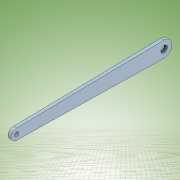
# Autodesk Inventor part: Transmision_Sup
Saved by Autodesk Inventor 2022 (Build 260153000, 153)
## iProperties
Created: 2022-02-14
Part Number: Transmision_Sup
Material: Genérico
Document SubType Name: Modeling
Designer: Marco
Density: 1 g/cm^3
Appearance: Azul acero
Author: Marco
Autodesk Inventor part; units mm, degrees
ref_plane "YZ Plane" through (0, 0, 0) normal (1, 0, 0) x (0, 1, 0)
ref_plane "XZ Plane" through (0, 0, 0) normal (0, 1, 0) x (-1, 0, 0)
ref_plane "XY Plane" through (0, 0, 0) normal (0, 0, 1) x (1, 0, 0)
sketch "Boceto1" plane through (0, 0, 0) normal (1, 0, 0) x (0, 1, 0)
  circle A0 centre (0, 0) radius 2
  arc A1 (5, 0) -> (-5, 0) centre (0, 0) ccw
  circle A2 centre (0, -140) radius 3.175
  arc A3 (-7.4952, -139.7322) -> (7.4952, -139.7322) centre (0, -140) ccw
  line L0 (5, 0) -> (7.5, -140)
  line L1 (-5, 0) -> (-7.5, -140)
  dimension "d0" = 4
  dimension "d1" = 10
  dimension "d2" = 6.35
  dimension "d3" = 140
  dimension "d4" = 15
  constraints: 6 point on circle, 4 centre point, 4 end point, 4 horizontal alignment, 3 coincident, 2 point on line, 1 vertical alignment
  measures "d0" diameter of A0
  measures "d1" diameter of A1
  measures "d2" diameter of A2
  measures "d3" distance of A2.centre point (0, 0)
  measures "d4" diameter of A3
extrude "Extrusión1" add sketch "Boceto1" along normal blind 3
